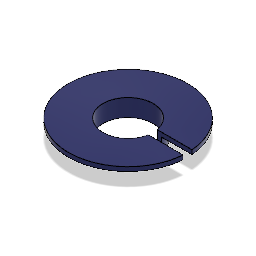
Collier feutre (Autodesk Fusion 360 design; units mm, degrees)
Autodesk Fusion 360 part; units mm, degrees
sketch "Sketch tranche" plane through (0, 0, 0) normal (0, 0, 1) x (1, 0, 0)
  line L0 (-13.6, 5) -> (-5.7, 5)
  line L1 (-5.7, 5) -> (-5.7, 4)
  line L2 (-5.7, 4) -> (-13.6, 4)
  line L3 (-13.6, 4) -> (-13.6, 5)
  line L4 (-5.7, 5) -> (-6.7, 5)
  line L5 (-6.7, 5) -> (-6.7, 1)
  line L6 (-6.7, 1) -> (-5.7, 1)
  line L7 (-5.7, 1) -> (-5.7, 5)
  dimension "d9" = 1
  dimension "d10" = 6.9
  dimension "d11" = 1
  dimension "d12" = 3
  dimension "d13" = 5.7
  constraint horizontal L0
  constraint vertical L1
  constraint horizontal L2
  constraint vertical L3
  constraint horizontal L4
  constraint vertical L5
  constraint horizontal L6
  constraint vertical L7
  measures "d9" distance of L0 L2
  measures "d10" distance of L3 L5
  measures "d11" distance of L1 L5
  measures "d12" distance of L2 L6
  measures "d13" horizontal distance of origin L6.end
revolve "Revolution tranche" add sketch "Sketch tranche" angle 360 about axis through (0, 1.75, 0) along (0, 1, 0)
sketch "Sketch6" plane through (0, 0, 0) normal (0, 1, 0) x (1, 0, 0)
  line L0 (5, -1) -> (14, -1)
  line L1 (14, -1) -> (14, 1)
  line L2 (14, 1) -> (5, 1)
  line L3 (5, 1) -> (5, -1)
  dimension "d14" = 9
  constraint horizontal L0
  constraint vertical L1
  constraint horizontal L2
  constraint vertical L3
  measures "d14" distance of L1 L3
extrude "Extrude découpe" cut sketch "Sketch6" along normal blind 8
named bodies: "Collier"
